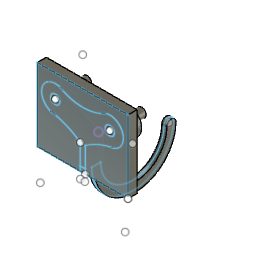
3D Plancha 3 (Autodesk Fusion 360 design; units mm, degrees)
Autodesk Fusion 360 part; units mm, degrees
sketch "Boceto1" plane through (0, 0, 0) normal (0, 0, 1) x (1, 0, 0)
sketch "Boceto2" plane through (0, 0, 0) normal (0, 1, 0) x (1, 0, 0)
  circle A0 centre (-6, -75) radius 1
  circle A1 centre (6, -75) radius 1
  arc A2 (5.0603, -77.849) -> (-4.904, -77.7926) centre (0.0291, -86.4912) ccw
  arc A3 (-7.0648, -72.1953) -> (-0.5128, -69.5) centre (-9.334, -57.368) ccw
  arc A4 (0.6137, -69.5) -> (6.7021, -72.0833) centre (9.3727, -57.323) ccw
  line L0 (-0.5, -69.5) -> (-0.5128, -69.5)
  arc A5 (-6.0328, -72.0002) -> (-4.325, -77.4888) centre (-6, -75) ccw
  arc A6 (4.2088, -77.4066) -> (6.4211, -72.0297) centre (6, -75) ccw
  line L1 (-10, -80) -> (10, -80)
  line L2 (-10, -80) -> (-10, -64)
  line L3 (-10, -64) -> (10, -64)
  line L4 (10, -80) -> (10, -64)
  line L5 (-0.5128, -69.5) -> (-0.5128, -64)
  line L6 (0.6137, -69.5) -> (0.6137, -64)
  line L7 (-0.5128, -65.0194) -> (0.6137, -65.0194)
  line L8 (-0.5, -62.5) -> (0.5, -62.5)
  dimension "d3" = 2
  dimension "d4" = 2
  dimension "d5" = 6
  dimension "d6" = 6
  dimension "d7" = 20
  dimension "d14" = 20
  dimension "d15" = 16
  dimension "d16" = 20
  dimension "d17" = 16
  constraint concentric A0 A5
  constraint concentric A1 A6
  constraint coincident A2.end A5
  constraint coincident A2.start A6
  constraint coincident A3.start A5
  constraint coincident A4.end A6
  constraint coincident A3 A5.start
  constraint coincident A2 A5.end
  constraint coincident A4 A6.end
  constraint coincident A2 A6.start
  constraint perpendicular L1 L2
  constraint perpendicular L2 L3
  constraint perpendicular L1 L4
  constraint coincident L3 L5.end
  constraint perpendicular L3 L5
  constraint coincident L5 L7.start
  constraint coincident L6 L7.end
  constraint perpendicular L6 L7
  constraint perpendicular L2 L8
  measures "d3" diameter of A0
  measures "d4" diameter of A1
  measures "d5" diameter of A5
  measures "d6" diameter of A6
  measures "d7" diameter of A2
  measures "d14" distance of L1.start L1.end
  measures "d15" distance of L1.start L2.end
  measures "d16" distance of L2.end L3.end
  measures "d17" distance of L1.end L3.end
extrude "Extruir1" add sketch "Boceto2" along normal blind 2 contours A2 A3 A4 A5 A6 L1 L2 L3 L4 L5 L6 makes body 1
extrude "Extruir2" add sketch "Boceto2" along normal blind 4 contours A2 A3 A4 A5 A6 L5 L6 L7 bodies 1
extrude "Extruir3" add sketch "Boceto2" along normal blind 7 contours A0 | A1 bodies 1
extrude "Extruir4" add sketch "Boceto2" along normal blind 4 contours L3 L5 L6 L7 bodies 1
sketch "Boceto3" plane through (0, 0, 0) normal (0, 1, 0) x (1, 0, 0)
sketch "Boceto4" plane through (0, 0, 0) normal (1, 0, 0) x (0, 1, 0)
  arc A0 (2, 64) -> (20, 64) centre (11, 64) ccw
  arc A1 (4, 64) -> (18, 64) centre (11, 64) ccw
  arc A2 (20, 64) -> (18, 64) centre (19, 64) ccw
  line L0 (4, 64) -> (2, 64)
  dimension "d26" = 18
  dimension "d27" = 14
  constraint concentric A0 A1
  constraint horizontal L0
  measures "d26" diameter of A0
  measures "d27" diameter of A1
extrude "Extruir5" add sketch "Boceto4" along normal blind 2 separate body makes body 2
move_body "Desplazar1" bodies 2 to x (1, 0, 0) y (0, 1, 0) z (0, 0, 1) at (-0.9372, 0, 0)
sketch "Boceto5" plane through (0, 4, 0) normal (0, 1, 0) x (-1, 0, 0)
  circle A0 centre (6, 75) radius 1
  circle A1 centre (-6, 75) radius 1
  arc A2 (7.0648, 72.1953) -> (4.904, 77.7926) centre (6, 75) ccw
  arc A3 (-5.0603, 77.849) -> (4.904, 77.7926) centre (-0.0291, 86.4912) ccw
  arc A4 (-5.0603, 77.849) -> (-6.7021, 72.0833) centre (-6, 75) ccw
  arc A5 (-0.6137, 69.5) -> (-6.7021, 72.0833) centre (-9.3727, 57.323) ccw
  line L0 (-0.6137, 69.5) -> (-0.6137, 64)
  line L1 (-0.6137, 64) -> (0.5128, 64)
  line L2 (0.5128, 64) -> (0.5128, 69.5)
  arc A6 (7.0648, 72.1953) -> (0.5128, 69.5) centre (9.334, 57.368) ccw
  point P0 (0.5, 69.5)
extrude "Extruir6" add sketch "Boceto4" along normal blind 1.114 separate body makes body 3
move_body "Desplazar2" bodies 3 to x (1, 0, 0) y (0, 1, 0) z (0, 0, 1) at (-0.5036, -0.0434, 0.0534)
hidden bodies 2
